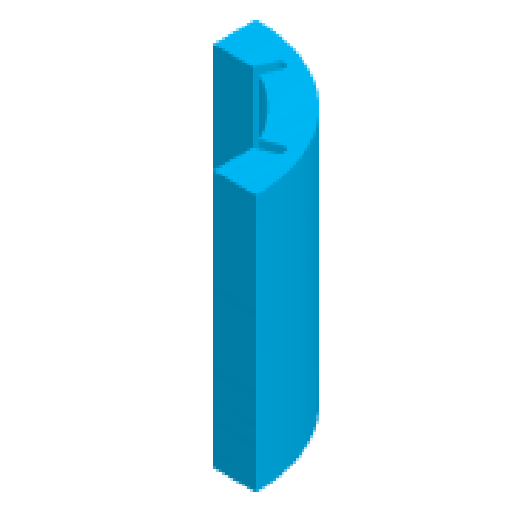
# Autodesk Inventor part: FoamPanel
Saved by Autodesk Inventor 2025.2 (Build 292293000, 293)
## iProperties
Created: 2024-11-16
Part Number: FoamPanel
Material: Generic
Document SubType Name: Modeling
Designer: alexb
Density: 1 g/cm^3
Appearance: Default
Author: alexb
Autodesk Inventor part; units mm, degrees
ref_plane "YZ Plane" through (0, 0, 0) normal (1, 0, 0) x (0, 1, 0)
ref_plane "XZ Plane" through (0, 0, 0) normal (0, 1, 0) x (-1, 0, 0)
ref_plane "XY Plane" through (0, 0, 0) normal (0, 0, 1) x (1, 0, 0)
sketch "Sketch1" plane through (0, 0, 0) normal (0, 1, 0) x (-1, 0, 0)
  arc A0 (-85, 0) -> (0, -85) centre (0, 0) ccw
  arc A1 (-70.3834, -25.9072) -> (-68.0877, -31.4494) centre (-69.291, -28.7013) ccw
  line L0 (0, 0) -> (-69.291, -28.7013) construction
  line L1 (-68.0877, -31.4494) -> (-58.8404, -27.619)
  line L2 (-70.3834, -25.9072) -> (-61.136, -22.0768)
  line L3 (0, 0) -> (-85, 0)
  arc A2 (-65, 0) -> (-61.136, -22.0768) centre (0, 0) ccw
  arc A3 (-58.8404, -27.619) -> (-27.619, -58.8404) centre (0, 0) ccw
  arc A4 (-22.0768, -61.136) -> (0, -65) centre (0, 0) ccw
  arc A5 (-75, 0) -> (0, -75) centre (0, 0) ccw
  line L4 (0, 0) -> (0, -85)
  line L5 (0, 0) -> (-28.7013, -69.291) construction
  arc A6 (-31.4494, -68.0877) -> (-25.9072, -70.3834) centre (-28.7013, -69.291) ccw
  line L6 (-25.9072, -70.3834) -> (-22.0768, -61.136)
  line L7 (-27.619, -58.8404) -> (-31.4494, -68.0877)
  line L8 (-22.0768, -61.136) -> (0, -61.136)
  line L9 (-61.136, -22.0768) -> (-61.136, 0)
  dimension "d20" = 75
  dimension "d11" = 6
  dimension "d16" = 22.5
  dimension "d19" = 20
  dimension "d21" = 45
  dimension "d22" = 85
  constraints: 20 end point, 12 point on circle, 6 centre point, 4 coincident, 4 point on line, 3 equal radius, 3 parallel, 2 equal length, 2 perpendicular, 1 horizontal, 1 vertical, 11 other
  measures "d11" diameter of A1
  measures "d16" angle of L3 L0
  measures "d19" radial gap between concentric circles of A0 A3
  measures "d21" angle of L0 L5
  measures "d22" radius of A0
extrude "Extrusion1" add sketch "Sketch1" along normal blind 144 contours L3 A5 A1 A6 L4 A0 | L3 A2 L2 A5 | A5 L6 A4 L4 | L3 L9 A2 | A4 L8 L4 | L1 A3 L7 A5
body "Solid1"
